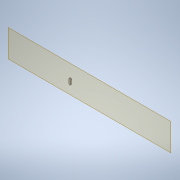
# Autodesk Inventor part: zaslepka_sruby_2
Saved by Autodesk Inventor 2022.3 (Build 263350000, 350)
## iProperties
Created: 2022-10-28
Part Number: zaslepka_sruby_2
Material: Generic
Document SubType Name: Modeling
Designer: komputer
Density: 1 g/cm^3
Appearance: Default
Author: komputer
Autodesk Inventor part; units mm, degrees
ref_plane "YZ Plane" through (0, 0, 0) normal (1, 0, 0) x (0, 1, 0)
ref_plane "XZ Plane" through (0, 0, 0) normal (0, 1, 0) x (-1, 0, 0)
ref_plane "XY Plane" through (0, 0, 0) normal (0, 0, 1) x (1, 0, 0)
ref_plane "Work Plane1" through (0, 0, 0) normal (0, 0, 1) x (1, 0, 0)
sketch "Sketch1" plane through (0, 0, 0) normal (0, 0, 1) x (1, 0, 0)
  line L0 (227.5976, -2) -> (227.5976, -22) projected
  arc A0 (217.5976, -22) -> (227.5976, -22) centre (222.5976, -22) ccw projected
  line L1 (217.5976, -22) -> (217.5976, -2) projected
  arc A1 (227.5976, -2) -> (217.5976, -2) centre (222.5976, -2) ccw projected
  line L2 (78.8821, -22) -> (78.8821, -2) projected
  arc A2 (88.8821, -2) -> (78.8821, -2) centre (83.8821, -2) ccw projected
  line L3 (88.8821, -2) -> (88.8821, -22) projected
  arc A3 (78.8821, -22) -> (88.8821, -22) centre (83.8821, -22) ccw projected
  line L4 (-82.1032, -2) -> (-82.1032, -22) projected
  arc A4 (-92.1032, -22) -> (-82.1032, -22) centre (-87.1032, -22) ccw projected
  line L5 (-92.1032, -22) -> (-92.1032, -2) projected
  arc A5 (-82.1032, -2) -> (-92.1032, -2) centre (-87.1032, -2) ccw projected
  line L6 (374.3969, 34.0458) -> (374.3969, -61) projected
  line L7 (344.0734, 61) -> (374.3969, 34.0458) projected
  line L8 (-316.3526, 61) -> (344.0734, 61) projected
  line L9 (-354.2917, 27.0499) -> (-316.3526, 61) projected
  line L10 (-54.9688, -61) -> (-354.2917, 27.0499) projected
  line L11 (374.3969, -61) -> (-54.9688, -61) projected
  line L12 (-87.1032, -22) -> (-87.1032, -2) construction
  line L13 (-82.2532, -22) -> (-82.2532, -2)
  line L14 (-91.9532, -2) -> (-91.9532, -22)
  arc A6 (-91.9532, -22) -> (-82.2532, -22) centre (-87.1032, -22) ccw
  arc A7 (-82.2532, -2) -> (-91.9532, -2) centre (-87.1032, -2) ccw
  line L15 (-87.1032, 3) -> (-87.1032, 2)
  line L16 (-87.1032, 2) -> (-84.3605, 2)
  line L17 (-87.1032, 2) -> (-89.8459, 2)
  line L18 (-87.1032, 2) -> (-88.6032, 2)
  line L19 (-88.6032, 2) -> (-85.6032, 2)
  line L20 (-85.6032, 2) -> (-85.6032, 4.0639)
  line L21 (-88.6032, 2) -> (-88.6032, 3.4505)
  point P0 (0, 0)
  point P1 (-87.1032, -12)
  point P2 (-85.6032, 2.6122)
  point P3 (-88.6032, 2.6122)
  dimension "d0" = 9.7
  dimension "d1" = 1
  dimension "d2" = 1.5
  dimension "d3" = 3
  constraints: 22 end point, 7 point on circle, 4 tangent, 3 point on line, 3 vertical, 2 centre point, 2 perpendicular, 1 midpoint, 1 parallel
  measures "d0" diameter of A7
  measures "d1" distance of L15.start L15.end
  measures "d2" distance of L15.end L18.end
  measures "d3" distance of L18.end L19.end
extrude "Extrusion1" add sketch "Sketch1" against normal blind 4 contours A7 L16 L20 | A7 L13 A6 L14 L17 L16 | L21 L17 A7
body "Solid1"
